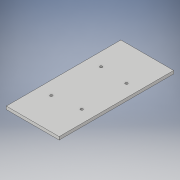
# Autodesk Inventor part: realsenses_plate
Saved by Autodesk Inventor 2019 (Build 230136000, 136)
## iProperties
Created: 2021-06-11
Part Number: realsenses_plate
Material: Типовые
Document SubType Name: Modeling
Designer: Петров Иван
Density: 1 g/cm^3
Appearance: По умолчанию
Author: Петров Иван
Autodesk Inventor part; units mm, degrees
ref_plane "YZ Plane" through (0, 0, 0) normal (1, 0, 0) x (0, 1, 0)
ref_plane "XZ Plane" through (0, 0, 0) normal (0, 1, 0) x (-1, 0, 0)
ref_plane "XY Plane" through (0, 0, 0) normal (0, 0, 1) x (1, 0, 0)
sketch "Sketch1" plane through (0, 0, 0) normal (0, 1, 0) x (-1, 0, 0)
  spline S0 degree 3 poles (-32.404854, -32.853236) (-32.408213, -32.73595) (-32.409911, -32.618547) (-32.409934, -32.501343) (-32.409955, -32.397684) (-32.409974, -32.293904) (-32.409993, -32.190169) (-32.410033, -31.969146) (-32.41007, -31.748122) (-32.410103, -31.527098) (-32.41017, -31.085051) (-32.410223, -30.643004) (-32.410266, -30.200957) (-32.410352, -29.316862) (-32.410395, -28.432768) (-32.410416, -27.548673) (-32.410444, -26.388246) (-32.410435, -25.228046) (-32.410446, -24.067555) (-32.410451, -23.45976) (-32.410462, -22.851867) (-32.410477, -22.244105) (-32.410527, -20.157589) (-32.410619, -18.070753) (-32.410664, -15.984323) (-32.410696, -14.53452) (-32.410704, -13.084832) (-32.410706, -11.63497) (-32.410708, -10.42824) (-32.410705, -9.226696) (-32.410708, -8.025862) (-32.410715, -5.363664) (-32.410749, -2.704993) (-32.410749, 0) (-32.410749, 2.70077) (-32.410715, 5.359553) (-32.410708, 8.025862) (-32.410707, 8.544603) (-32.410707, 9.06363) (-32.410707, 9.583301) (-32.410707, 11.716216) (-32.41071, 13.850051) (-32.410664, 15.984323) (-32.410606, 18.679415) (-32.41047, 21.375766) (-32.410446, 24.067555) (-32.410425, 26.312694) (-32.410471, 28.55511) (-32.410201, 30.801569) (-32.410148, 31.243615) (-32.410083, 31.685661) (-32.410004, 32.127707) (-32.409982, 32.252247) (-32.409959, 32.376902) (-32.409934, 32.501343) (-32.409915, 32.59775) (-32.408764, 32.694267) (-32.406487, 32.790697) (-32.401273, 33.0116) (-32.390165, 33.232367) (-32.373199, 33.452997) (-32.339266, 33.894259) (-32.28153, 34.337158) (-32.200857, 34.773898) (-32.120183, 35.210638) (-32.017096, 35.639812) (-31.892023, 36.061563) (-31.803491, 36.360098) (-31.703903, 36.654969) (-31.593121, 36.94617) (-31.39089, 37.477752) (-31.151562, 37.997105) (-30.875182, 38.502046) (-30.760914, 38.710811) (-30.641216, 38.915391) (-30.516203, 39.115805) (-30.173207, 39.665673) (-29.790661, 40.184302) (-29.36895, 40.672553) (-29.245622, 40.81534) (-29.118935, 40.95548) (-28.988811, 41.092954) (-28.815373, 41.276189) (-28.635833, 41.454691) (-28.450153, 41.628366) (-28.125165, 41.932343) (-27.784487, 42.218481) (-27.432415, 42.483881) (-27.308772, 42.577086) (-27.18357, 42.667861) (-27.056809, 42.756201) (-26.46167, 43.170951) (-25.83254, 43.532746) (-25.16884, 43.840615) (-25.051477, 43.895056) (-24.933051, 43.94777) (-24.813786, 43.998631) (-24.523994, 44.122212) (-24.22923, 44.2348) (-23.933007, 44.33546) (-23.514871, 44.477546) (-23.091358, 44.596955) (-22.662502, 44.693838) (-22.570374, 44.714651) (-22.477996, 44.734419) (-22.38537, 44.753136) (-22.046825, 44.821544) (-21.70496, 44.875937) (-21.359741, 44.916201) (-20.920071, 44.967482) (-20.473811, 44.995783) (-20.027865, 45) knots 0 0 0 0 0.00414579 0.00414579 0.00414579 0.0078125 0.0078125 0.0078125 0.015625 0.015625 0.015625 0.03125 0.03125 0.03125 0.0625 0.0625 0.0625 0.1035175 0.1035175 0.1035175 0.125 0.125 0.125 0.19875187 0.19875187 0.19875187 0.25 0.25 0.25 0.29265414 0.29265414 0.29265414 0.38721651 0.38721651 0.38721651 0.48163124 0.48163124 0.48163124 0.5 0.5 0.5 0.57539191 0.57539191 0.57539191 0.67059447 0.67059447 0.67059447 0.75 0.75 0.75 0.765625 0.765625 0.765625 0.77002712 0.77002712 0.77002712 0.7734375 0.7734375 0.7734375 0.78125 0.78125 0.78125 0.796875 0.796875 0.796875 0.8125 0.8125 0.8125 0.82356007 0.82356007 0.82356007 0.84375 0.84375 0.84375 0.85209742 0.85209742 0.85209742 0.875 0.875 0.875 0.88169776 0.88169776 0.88169776 0.890625 0.890625 0.890625 0.90625 0.90625 0.90625 0.91173731 0.91173731 0.91173731 0.9375 0.9375 0.9375 0.94205566 0.94205566 0.94205566 0.953125 0.953125 0.953125 0.96875 0.96875 0.96875 0.97210662 0.97210662 0.97210662 0.984375 0.984375 0.984375 1 1 1 1
  spline S1 degree 3 poles (-28.410193, 32.5) (-28.410193, 33.765572) (-28.133676, 34.931308) (-27.671254, 35.965522) (-27.208832, 36.999736) (-26.560504, 37.902428) (-25.780808, 38.647111) (-25.001113, 39.391795) (-24.090049, 39.97847) (-23.095481, 40.380521) (-22.100912, 40.782573) (-21.02284, 41) (-19.910193, 41) (-18.797545, 41) (-17.719473, 40.782573) (-16.724904, 40.380521) (-15.730336, 39.97847) (-14.819272, 39.391795) (-14.039577, 38.647111) (-13.259881, 37.902428) (-12.611553, 36.999736) (-12.149131, 35.965522) (-11.686709, 34.931308) (-11.410193, 33.765572) (-11.410193, 32.5) knots 0 0 0 0 0.125 0.125 0.125 0.25 0.25 0.25 0.375 0.375 0.375 0.5 0.5 0.5 0.625 0.625 0.625 0.75 0.75 0.75 0.875 0.875 0.875 1 1 1 1
  line L0 (-28.410193, -32.5) -> (-28.410193, 32.5)
  line L1 (-11.410193, 32.5) -> (-11.410193, -9.130692)
  line L2 (-11.410193, -9.130692) -> (-11.410193, -32.5)
  spline S2 degree 3 poles (-11.92122, -35.403236) (-11.99101, -35.594681) (-12.067149, -35.782168) (-12.149131, -35.965522) (-12.611553, -36.999736) (-13.259881, -37.902428) (-14.039577, -38.647111) (-14.819272, -39.391795) (-15.730336, -39.97847) (-16.724904, -40.380521) (-17.719473, -40.782573) (-18.797545, -41) (-19.910193, -41) (-21.02284, -41) (-22.100912, -40.782573) (-23.095481, -40.380521) (-24.090049, -39.97847) (-25.001113, -39.391795) (-25.780808, -38.647111) (-26.560504, -37.902428) (-27.208832, -36.999736) (-27.671254, -35.965522) (-27.753236, -35.782168) (-27.829375, -35.594681) (-27.899165, -35.403236) knots 0.102839 0.102839 0.102839 0.102839 0.125 0.125 0.125 0.25 0.25 0.25 0.375 0.375 0.375 0.5 0.5 0.5 0.625 0.625 0.625 0.75 0.75 0.75 0.875 0.875 0.875 0.897161 0.897161 0.897161 0.897161
  ellipse E0 centre (-27.409985, -30.903735) end of major axis (-43.224744, -27.538991) minor radius 11.659046 (-11.885471, -35.303236) -> (-11.410193, -32.5) ccw
  ellipse E1 centre (-12.410416, -30.903738) end of major axis (-28.225158, -34.268479) minor radius 11.659041 (-28.410193, -32.5) -> (-27.934914, -35.303236) ccw
  spline S3 degree 3 poles (-20.135916, -44.926171) (-20.902232, -44.912188) (-21.656156, -44.828474) (-22.39639, -44.67772) (-22.948546, -44.56527) (-23.493405, -44.415278) (-24.031365, -44.226793) (-24.310103, -44.129132) (-24.58603, -44.021306) (-24.856048, -43.904514) (-24.890974, -43.889408) (-24.925802, -43.874152) (-24.960525, -43.858751) (-25.263696, -43.724284) (-25.560172, -43.578241) (-25.850131, -43.420931) (-26.291576, -43.181437) (-26.717955, -42.915946) (-27.128881, -42.623661) (-27.257781, -42.531977) (-27.385148, -42.437641) (-27.510974, -42.340653) (-27.774451, -42.137563) (-28.031837, -41.922148) (-28.278086, -41.698847) (-28.524335, -41.475546) (-28.760531, -41.243618) (-28.986777, -41.003148) (-29.015281, -40.972852) (-29.043627, -40.942419) (-29.071813, -40.911851) (-29.491074, -40.457166) (-29.875526, -39.972573) (-30.22442, -39.457475) (-30.348377, -39.274468) (-30.468123, -39.087073) (-30.582688, -38.896485) (-30.640191, -38.800823) (-30.696393, -38.704359) (-30.751212, -38.60729) (-30.915247, -38.316831) (-31.066945, -38.021018) (-31.206902, -37.720112) (-31.358831, -37.393466) (-31.497133, -37.060343) (-31.621381, -36.721723) (-31.726048, -36.436468) (-31.82072, -36.147348) (-31.905041, -35.853236) knots 0 0 0 0 0.14319106 0.14319106 0.14319106 0.25 0.25 0.25 0.30534172 0.30534172 0.30534172 0.3125 0.3125 0.3125 0.375 0.375 0.375 0.47015259 0.47015259 0.47015259 0.5 0.5 0.5 0.5625 0.5625 0.5625 0.625 0.625 0.625 0.63287425 0.63287425 0.63287425 0.75 0.75 0.75 0.7916132 0.7916132 0.7916132 0.8125 0.8125 0.8125 0.875 0.875 0.875 0.94284614 0.94284614 0.94284614 1 1 1 1
  ellipse E2 centre (-27.409985, -30.903735) end of major axis (-43.224744, -27.538991) minor radius 11.659046 (-11.885471, -35.303236) -> (-11.410193, -32.5) ccw
  line L3 (-11.410193, -9.130692) -> (-11.410193, -32.5)
  line L4 (-11.410193, 32.5) -> (-11.410193, -9.130692)
  spline S4 degree 3 poles (-28.410193, 32.5) (-28.410193, 33.765572) (-28.133677, 34.931308) (-27.671254, 35.965522) (-27.208832, 36.999736) (-26.560504, 37.902428) (-25.780809, 38.647111) (-25.001113, 39.391795) (-24.090049, 39.97847) (-23.095481, 40.380521) (-22.100913, 40.782573) (-21.02284, 41) (-19.910193, 41) (-18.797545, 41) (-17.719473, 40.782573) (-16.724904, 40.380521) (-15.730336, 39.97847) (-14.819273, 39.391795) (-14.039577, 38.647111) (-13.259881, 37.902428) (-12.611553, 36.999736) (-12.149131, 35.965522) (-11.686709, 34.931308) (-11.410193, 33.765572) (-11.410193, 32.5) knots 0 0 0 0 0.125 0.125 0.125 0.25 0.25 0.25 0.375 0.375 0.375 0.5 0.5 0.5 0.625 0.625 0.625 0.75 0.75 0.75 0.875 0.875 0.875 1 1 1 1
  line L5 (-28.410193, -32.5) -> (-28.410193, 32.5)
  ellipse E3 centre (-12.410416, -30.903738) end of major axis (-28.225158, -34.268479) minor radius 11.659041 (-28.410193, -32.5) -> (-27.934914, -35.303236) ccw
  circle A0 centre (-19.910193, 22.5) radius 1.25
  circle A1 centre (-19.910193, -22.5) radius 1.25
  spline S5 degree 3 poles (-7.409638, -8.902626) (-7.409642, -11.263271) (-7.409635, -13.623588) (-7.409688, -15.984285) (-7.409726, -17.615445) (-7.409792, -19.246809) (-7.409843, -20.877933) (-7.409877, -21.941017) (-7.409905, -23.004462) (-7.409916, -24.06752) (-7.409926, -25.000298) (-7.409923, -25.932787) (-7.409937, -26.865587) (-7.409952, -27.863529) (-7.409987, -28.861472) (-7.410072, -29.859414) (-7.410115, -30.358385) (-7.410171, -30.857356) (-7.410243, -31.356327) (-7.410279, -31.605813) (-7.410319, -31.855298) (-7.410363, -32.104784) (-7.410387, -32.236971) (-7.410411, -32.369257) (-7.410437, -32.501339) (-7.410461, -32.618544) (-7.412158, -32.735941) (-7.415518, -32.853236) knots 0 0 0 0 0.29568906 0.29568906 0.29568906 0.5 0.5 0.5 0.6331595 0.6331595 0.6331595 0.75 0.75 0.75 0.875 0.875 0.875 0.9375 0.9375 0.9375 0.96875 0.96875 0.96875 0.98530746 0.98530746 0.98530746 1 1 1 1
  spline S6 degree 3 poles (-7.409638, -8.902626) (-7.398668, -9.006825) (-9.14047, -8.698904) (-11.410193, -9.130692) knots 0 0 0 0 1 1 1 1
  line L6 (-11.410193, -9.130692) -> (-11.410193, -32.5)
  ellipse E4 centre (-27.409985, -30.903735) end of major axis (-43.224744, -27.538991) minor radius 11.659046 (-11.885471, -35.303236) -> (-11.410193, -32.5) ccw
  line L7 (-11.885471, -35.303236) -> (-7.757702, -35.303236)
  spline S7 degree 3 poles (-7.757702, -35.303236) (-7.758844, -35.303236) (-7.761073, -35.30773) (-7.767821, -35.325968) (-7.772438, -35.340145) (-7.78659, -35.386369) (-7.797308, -35.423345) (-7.823066, -35.51376) (-7.838041, -35.566981) (-7.866767, -35.668696) (-7.879817, -35.714794) (-7.897842, -35.778081) (-7.902464, -35.794277) (-7.90927, -35.818079) (-7.911434, -35.825641) (-7.915514, -35.839882) (-7.917428, -35.846559) (-7.919345, -35.853236) knots 0 0 0 0 0.13804482 0.13804482 0.28388387 0.28388387 0.50004609 0.50004609 0.72328448 0.72328448 0.89210226 0.89210226 0.94966157 0.94966157 0.97641027 0.97641027 1 1 1 1
  spline S8 degree 3 poles (-7.919345, -35.853236) (-8.003152, -36.145286) (-8.097043, -36.431979) (-8.200582, -36.714498) (-8.328208, -37.062745) (-8.47045, -37.404583) (-8.626747, -37.739075) (-8.810346, -38.131998) (-9.013716, -38.515699) (-9.237855, -38.889015) (-9.35932, -39.09132) (-9.486915, -39.290583) (-9.620818, -39.486955) (-9.811316, -39.766324) (-10.014117, -40.038912) (-10.225707, -40.300477) (-10.393712, -40.508163) (-10.567792, -40.709695) (-10.747887, -40.905165) (-10.794607, -40.955875) (-10.841734, -41.006176) (-10.889261, -41.056069) (-11.350717, -41.540498) (-11.849576, -41.987112) (-12.386918, -42.394816) (-12.486805, -42.470605) (-12.588167, -42.545124) (-12.690734, -42.618124) (-12.864047, -42.741476) (-13.040808, -42.860477) (-13.219487, -42.974259) (-13.503909, -43.155378) (-13.7942, -43.324035) (-14.090213, -43.480544) (-14.376118, -43.631709) (-14.667362, -43.771537) (-14.964004, -43.8999) (-15.281618, -44.037338) (-15.605429, -44.161639) (-15.935451, -44.272737) (-16.254577, -44.380167) (-16.581053, -44.475594) (-16.9089, -44.557066) (-17.080253, -44.599649) (-17.251997, -44.638463) (-17.424125, -44.673526) (-17.581326, -44.705549) (-17.738847, -44.734442) (-17.896686, -44.760264) (-18.558021, -44.868455) (-19.224843, -44.923373) (-19.897251, -44.924079) (-19.901566, -44.924083) (-19.90588, -44.924086) (-19.910193, -44.924086) (-20.241963, -44.924086) (-20.576611, -44.910627) (-20.909693, -44.883796) (-21.247106, -44.856615) (-21.5813, -44.815961) (-21.912343, -44.762119) (-22.074408, -44.73576) (-22.235717, -44.706233) (-22.39627, -44.673528) (-22.891627, -44.572622) (-23.379775, -44.441685) (-23.860799, -44.280846) (-24.196316, -44.16866) (-24.529506, -44.041364) (-24.856421, -43.899904) (-25.150109, -43.772821) (-25.438729, -43.634322) (-25.719775, -43.486069) (-26.209658, -43.227655) (-26.679695, -42.938431) (-27.129738, -42.618131) (-27.225287, -42.550128) (-27.319927, -42.480713) (-27.41366, -42.409893) (-27.948886, -42.0055) (-28.458682, -41.551215) (-28.922894, -41.064862) (-28.973321, -41.01203) (-29.02324, -40.9588) (-29.072649, -40.905176) (-29.478082, -40.465148) (-29.849491, -39.998649) (-30.186959, -39.505722) (-30.324635, -39.304624) (-30.456615, -39.099116) (-30.58276, -38.889029) (-30.630057, -38.810259) (-30.676532, -38.730845) (-30.722184, -38.6508) (-30.889595, -38.357265) (-31.045877, -38.05518) (-31.189193, -37.749189) (-31.347794, -37.410564) (-31.491558, -37.065293) (-31.620128, -36.714515) (-31.723916, -36.431349) (-31.817776, -36.144633) (-31.901409, -35.853236) knots 0 0 0 0 0.02799367 0.02799367 0.02799367 0.0625 0.0625 0.0625 0.10303401 0.10303401 0.10303401 0.125 0.125 0.125 0.15625 0.15625 0.15625 0.18106293 0.18106293 0.18106293 0.1875 0.1875 0.1875 0.25 0.25 0.25 0.26161819 0.26161819 0.26161819 0.28125 0.28125 0.28125 0.3125 0.3125 0.3125 0.34268303 0.34268303 0.34268303 0.375 0.375 0.375 0.40625 0.40625 0.40625 0.42258324 0.42258324 0.42258324 0.4375 0.4375 0.4375 0.5 0.5 0.5 0.50040103 0.50040103 0.50040103 0.53125 0.53125 0.53125 0.5625 0.5625 0.5625 0.57779868 0.57779868 0.57779868 0.625 0.625 0.625 0.65792316 0.65792316 0.65792316 0.6875 0.6875 0.6875 0.7390545 0.7390545 0.7390545 0.75 0.75 0.75 0.8125 0.8125 0.8125 0.81928929 0.81928929 0.81928929 0.875 0.875 0.875 0.89772826 0.89772826 0.89772826 0.90625 0.90625 0.90625 0.9375 0.9375 0.9375 0.97208291 0.97208291 0.97208291 1 1 1 1
  spline S9 degree 3 poles (-31.901409, -35.853236) (-31.903324, -35.846565) (-31.905236, -35.839895) (-31.909312, -35.82567) (-31.911474, -35.818117) (-31.918271, -35.79435) (-31.922886, -35.778181) (-31.940872, -35.715036) (-31.953892, -35.669047) (-31.982604, -35.567376) (-31.997591, -35.514102) (-32.023361, -35.423609) (-32.034081, -35.386601) (-32.048248, -35.340272) (-32.052873, -35.326045) (-32.05963, -35.307745) (-32.061857, -35.303236) (-32.062995, -35.303236) knots 0 0 0 0 0.02356692 0.02356692 0.05028405 0.05028405 0.10774901 0.10774901 0.27614786 0.27614786 0.49948807 0.49948807 0.71561552 0.71561552 0.86172473 0.86172473 1 1 1 1
  line L8 (-32.062995, -35.303236) -> (-27.934914, -35.303236)
  ellipse E5 centre (-12.410416, -30.903738) end of major axis (-28.225158, -34.268479) minor radius 11.659041 (-28.410193, -32.5) -> (-27.934914, -35.303236) ccw
  line L9 (-28.410193, -32.5) -> (-28.410193, 32.5)
  spline S10 degree 3 poles (-28.410193, 32.5) (-28.410193, 33.765572) (-28.133676, 34.931308) (-27.671254, 35.965522) (-27.208832, 36.999736) (-26.560504, 37.902428) (-25.780808, 38.647111) (-25.001113, 39.391795) (-24.090049, 39.97847) (-23.095481, 40.380521) (-22.100912, 40.782573) (-21.02284, 41) (-19.910193, 41) (-18.797545, 41) (-17.719473, 40.782573) (-16.724904, 40.380521) (-15.730336, 39.97847) (-14.819272, 39.391795) (-14.039577, 38.647111) (-13.259881, 37.902428) (-12.611553, 36.999736) (-12.149131, 35.965522) (-11.686709, 34.931308) (-11.410193, 33.765572) (-11.410193, 32.5) knots 0 0 0 0 0.125 0.125 0.125 0.25 0.25 0.25 0.375 0.375 0.375 0.5 0.5 0.5 0.625 0.625 0.625 0.75 0.75 0.75 0.875 0.875 0.875 1 1 1 1
  line L10 (-11.410193, 32.5) -> (-11.410193, -9.130692)
  spline S11 degree 3 poles (-7.409638, -8.902626) (-7.408932, -8.899194) (-7.41554, -8.881327) (-7.442844, -8.816766) (-7.463738, -8.769717) (-7.536437, -8.603714) (-7.599257, -8.458754) (-7.724577, -8.122213) (-7.786434, -7.935427) (-7.879306, -7.556662) (-7.913159, -7.371174) (-7.937278, -7.119769) (-7.941464, -7.06115) (-7.945382, -6.9757) (-7.946297, -6.949166) (-7.947438, -6.899489) (-7.947739, -6.876366) (-7.947807, -6.853236) knots 0 0 0 0 0.13056971 0.13056971 0.2645065 0.2645065 0.49982844 0.49982844 0.71627112 0.71627112 0.89885892 0.89885892 0.95382194 0.95382194 0.9785172 0.9785172 1 1 1 1
  spline S12 degree 3 poles (-7.947807, -6.853236) (-7.954633, -4.568884) (-7.957468, -2.286953) (-7.957468, 0) (-7.957468, 2.385018) (-7.954386, 4.76446) (-7.946908, 7.146764) knots 0 0 0 0 0.48950496 0.48950496 0.48950496 1 1 1 1
  spline S13 degree 3 poles (-7.946908, 7.146764) (-7.946835, 7.169899) (-7.946531, 7.193028) (-7.945383, 7.242716) (-7.944465, 7.269255) (-7.940538, 7.354723) (-7.936347, 7.413355) (-7.912212, 7.66482) (-7.878365, 7.850357) (-7.785562, 8.229172) (-7.723783, 8.415967) (-7.598689, 8.752471) (-7.536024, 8.897388) (-7.46354, 9.063319) (-7.442718, 9.110341) (-7.415511, 9.174866) (-7.408931, 9.192724) (-7.409638, 9.196154) knots 0 0 0 0 0.02148885 0.02148885 0.04619107 0.04619107 0.10116958 0.10116958 0.28381522 0.28381522 0.50028176 0.50028176 0.73556793 0.73556793 0.86946283 0.86946283 1 1 1 1
  ellipse E6 centre (-19.910191, 45) end of major axis (-20.032475, 45) minor radius 0 (-20.027865, 45) -> (-19.792521, 45) ccw
  spline S14 degree 3 poles (-32.404854, -32.853236) (-32.408213, -32.73595) (-32.409911, -32.618547) (-32.409934, -32.501343) (-32.409955, -32.397684) (-32.409974, -32.293904) (-32.409993, -32.190169) (-32.410033, -31.969146) (-32.41007, -31.748122) (-32.410103, -31.527098) (-32.41017, -31.085051) (-32.410223, -30.643004) (-32.410266, -30.200957) (-32.410352, -29.316862) (-32.410395, -28.432768) (-32.410416, -27.548673) (-32.410444, -26.388246) (-32.410435, -25.228046) (-32.410446, -24.067555) (-32.410451, -23.45976) (-32.410462, -22.851867) (-32.410477, -22.244105) (-32.410527, -20.157589) (-32.410619, -18.070753) (-32.410664, -15.984323) (-32.410696, -14.53452) (-32.410704, -13.084832) (-32.410706, -11.63497) (-32.410708, -10.42824) (-32.410705, -9.226696) (-32.410708, -8.025862) (-32.410715, -5.363664) (-32.410749, -2.704993) (-32.410749, 0) (-32.410749, 2.70077) (-32.410715, 5.359553) (-32.410708, 8.025862) (-32.410707, 8.544603) (-32.410707, 9.06363) (-32.410707, 9.583301) (-32.410707, 11.716216) (-32.41071, 13.850051) (-32.410664, 15.984323) (-32.410606, 18.679415) (-32.41047, 21.375766) (-32.410446, 24.067555) (-32.410425, 26.312694) (-32.410471, 28.55511) (-32.410201, 30.801569) (-32.410148, 31.243615) (-32.410083, 31.685661) (-32.410004, 32.127707) (-32.409982, 32.252247) (-32.409959, 32.376902) (-32.409934, 32.501343) (-32.409915, 32.59775) (-32.408764, 32.694267) (-32.406487, 32.790697) (-32.401273, 33.0116) (-32.390165, 33.232367) (-32.373199, 33.452997) (-32.339266, 33.894259) (-32.28153, 34.337158) (-32.200857, 34.773898) (-32.120183, 35.210638) (-32.017096, 35.639812) (-31.892023, 36.061563) (-31.803491, 36.360098) (-31.703903, 36.654969) (-31.593121, 36.94617) (-31.39089, 37.477752) (-31.151562, 37.997105) (-30.875182, 38.502046) (-30.760914, 38.710811) (-30.641216, 38.915391) (-30.516203, 39.115805) (-30.173207, 39.665673) (-29.790661, 40.184302) (-29.36895, 40.672553) (-29.245622, 40.81534) (-29.118935, 40.95548) (-28.988811, 41.092954) (-28.815373, 41.276189) (-28.635833, 41.454691) (-28.450153, 41.628366) (-28.125165, 41.932343) (-27.784487, 42.218481) (-27.432415, 42.483881) (-27.308772, 42.577086) (-27.18357, 42.667861) (-27.056809, 42.756201) (-26.46167, 43.170951) (-25.83254, 43.532746) (-25.16884, 43.840615) (-25.051477, 43.895056) (-24.933051, 43.94777) (-24.813786, 43.998631) (-24.523994, 44.122212) (-24.22923, 44.2348) (-23.933007, 44.33546) (-23.514871, 44.477546) (-23.091358, 44.596955) (-22.662502, 44.693838) (-22.570374, 44.714651) (-22.477996, 44.734419) (-22.38537, 44.753136) (-22.046825, 44.821544) (-21.70496, 44.875937) (-21.359741, 44.916201) (-20.920071, 44.967482) (-20.473811, 44.995783) (-20.027865, 45) knots 0 0 0 0 0.00414579 0.00414579 0.00414579 0.0078125 0.0078125 0.0078125 0.015625 0.015625 0.015625 0.03125 0.03125 0.03125 0.0625 0.0625 0.0625 0.1035175 0.1035175 0.1035175 0.125 0.125 0.125 0.19875187 0.19875187 0.19875187 0.25 0.25 0.25 0.29265414 0.29265414 0.29265414 0.38721651 0.38721651 0.38721651 0.48163124 0.48163124 0.48163124 0.5 0.5 0.5 0.57539191 0.57539191 0.57539191 0.67059447 0.67059447 0.67059447 0.75 0.75 0.75 0.765625 0.765625 0.765625 0.77002712 0.77002712 0.77002712 0.7734375 0.7734375 0.7734375 0.78125 0.78125 0.78125 0.796875 0.796875 0.796875 0.8125 0.8125 0.8125 0.82356007 0.82356007 0.82356007 0.84375 0.84375 0.84375 0.85209742 0.85209742 0.85209742 0.875 0.875 0.875 0.88169776 0.88169776 0.88169776 0.890625 0.890625 0.890625 0.90625 0.90625 0.90625 0.91173731 0.91173731 0.91173731 0.9375 0.9375 0.9375 0.94205566 0.94205566 0.94205566 0.953125 0.953125 0.953125 0.96875 0.96875 0.96875 0.97210662 0.97210662 0.97210662 0.984375 0.984375 0.984375 1 1 1 1
  spline S15 degree 3 poles (-32.326118, -33.903236) (-32.327007, -33.903236) (-32.328715, -33.895) (-32.333743, -33.861541) (-32.337123, -33.835589) (-32.347083, -33.749915) (-32.354346, -33.680402) (-32.369383, -33.51231) (-32.377025, -33.415241) (-32.389523, -33.2211) (-32.394565, -33.12798) (-32.399896, -33.000336) (-32.401115, -32.968405) (-32.402735, -32.921618) (-32.403222, -32.906877) (-32.404093, -32.879166) (-32.404483, -32.866202) (-32.404854, -32.853236) knots 0 0 0 0 0.13773636 0.13773636 0.28245528 0.28245528 0.4998262 0.4998262 0.71460149 0.71460149 0.89132086 0.89132086 0.94969153 0.94969153 0.97647884 0.97647884 1 1 1 1
  line L11 (-32.275001, -33.903236) -> (-32.326118, -33.903236)
  spline S16 degree 3 poles (-32.082303, -34.853236) (-32.084676, -34.841371) (-32.087042, -34.829506) (-32.09207, -34.804213) (-32.094728, -34.790789) (-32.103063, -34.748561) (-32.108688, -34.719844) (-32.130326, -34.608554) (-32.145652, -34.527896) (-32.178504, -34.352726) (-32.195119, -34.262366) (-32.224113, -34.107828) (-32.236352, -34.04447) (-32.25334, -33.965771) (-32.25917, -33.941768) (-32.268606, -33.91085) (-32.272281, -33.903236) (-32.275001, -33.903236) knots 0 0 0 0 0.02405151 0.02405151 0.0512956 0.0512956 0.10987642 0.10987642 0.27988487 0.27988487 0.49965886 0.49965886 0.71628377 0.71628377 0.86179308 0.86179308 1 1 1 1
  spline S17 degree 3 poles (-20.17139, -44.853236) (-20.878029, -44.838222) (-21.573226, -44.763643) (-22.257416, -44.631762) (-22.301762, -44.623215) (-22.346062, -44.614422) (-22.390317, -44.605384) (-23.028853, -44.474979) (-23.65793, -44.294096) (-24.276424, -44.061427) (-24.47081, -43.988301) (-24.66254, -43.910608) (-24.851638, -43.828396) (-25.305911, -43.630899) (-25.745054, -43.407502) (-26.16963, -43.159057) (-26.497285, -42.967327) (-26.816345, -42.760565) (-27.126353, -42.538413) (-27.385274, -42.35287) (-27.637877, -42.156573) (-27.883918, -41.949598) (-28.305343, -41.595087) (-28.698989, -41.216742) (-29.065485, -40.815445) (-29.16915, -40.701936) (-29.270623, -40.586577) (-29.369939, -40.469336) (-29.811526, -39.948054) (-30.211115, -39.389501) (-30.564084, -38.794047) (-30.571157, -38.782114) (-30.578212, -38.770167) (-30.585247, -38.758206) (-30.943356, -38.149318) (-31.244219, -37.518322) (-31.494339, -36.86773) (-31.525136, -36.787624) (-31.555162, -36.707173) (-31.584396, -36.626428) (-31.792589, -36.051387) (-31.960654, -35.461445) (-32.082303, -34.853236) knots 0 0 0 0 0.125 0.125 0.125 0.13310181 0.13310181 0.13310181 0.25 0.25 0.25 0.28673977 0.28673977 0.28673977 0.375 0.375 0.375 0.44311226 0.44311226 0.44311226 0.5 0.5 0.5 0.5974389 0.5974389 0.5974389 0.625 0.625 0.625 0.74754435 0.74754435 0.74754435 0.75 0.75 0.75 0.875 0.875 0.875 0.89039091 0.89039091 0.89039091 1 1 1 1
  line L12 (-20.17139, -44.853236) -> (-19.649008, -44.853236)
  spline S18 degree 3 poles (-7.738713, -34.853236) (-7.860311, -35.461404) (-8.028327, -36.051343) (-8.236488, -36.626409) (-8.265735, -36.707207) (-8.295776, -36.787711) (-8.326589, -36.867869) (-8.576705, -37.518543) (-8.877592, -38.149652) (-9.235782, -38.758677) (-9.242721, -38.770476) (-9.249678, -38.78226) (-9.256654, -38.79403) (-9.609761, -39.389781) (-10.009148, -39.948038) (-10.450617, -40.469231) (-10.549953, -40.586506) (-10.651446, -40.701897) (-10.755129, -40.815433) (-11.121335, -41.21644) (-11.514619, -41.594489) (-11.935591, -41.948716) (-12.181737, -42.155836) (-12.434737, -42.352496) (-12.69416, -42.538407) (-13.004032, -42.760472) (-13.323062, -42.967221) (-13.650378, -43.158779) (-14.075179, -43.40739) (-14.514473, -43.63087) (-14.9688, -43.828397) (-15.15761, -43.910486) (-15.349026, -43.988062) (-15.543071, -44.06108) (-16.161281, -44.293705) (-16.791217, -44.474918) (-17.430074, -44.605391) (-17.47426, -44.614415) (-17.518489, -44.623194) (-17.562759, -44.631729) (-18.247107, -44.763656) (-18.942379, -44.838234) (-19.649008, -44.853236) knots 0 0 0 0 0.10960083 0.10960083 0.10960083 0.125 0.125 0.125 0.25 0.25 0.25 0.25242164 0.25242164 0.25242164 0.375 0.375 0.375 0.4025818 0.4025818 0.4025818 0.5 0.5 0.5 0.55696145 0.55696145 0.55696145 0.625 0.625 0.625 0.71330281 0.71330281 0.71330281 0.75 0.75 0.75 0.86691377 0.86691377 0.86691377 0.875 0.875 0.875 1 1 1 1
  spline S19 degree 3 poles (-7.545928, -33.903236) (-7.548655, -33.903236) (-7.552333, -33.910824) (-7.561767, -33.941634) (-7.567592, -33.965551) (-7.584574, -34.044068) (-7.596815, -34.10737) (-7.625801, -34.261778) (-7.642403, -34.352049) (-7.675265, -34.527294) (-7.690621, -34.608135) (-7.712301, -34.719667) (-7.717932, -34.748431) (-7.726277, -34.790723) (-7.728938, -34.804162) (-7.733969, -34.829483) (-7.736337, -34.84136) (-7.738713, -34.853236) knots 0 0 0 0 0.13797105 0.13797105 0.28320611 0.28320611 0.49987241 0.49987241 0.71955484 0.71955484 0.88997298 0.88997298 0.94864929 0.94864929 0.97592532 0.97592532 1 1 1 1
  line L13 (-7.494451, -33.903236) -> (-7.545928, -33.903236)
  spline S20 degree 3 poles (-7.415518, -32.853236) (-7.415889, -32.866192) (-7.416279, -32.879146) (-7.417149, -32.906834) (-7.417636, -32.921561) (-7.419255, -32.968293) (-7.420473, -33.000185) (-7.425797, -33.127573) (-7.43083, -33.220493) (-7.443328, -33.414553) (-7.450985, -33.51171) (-7.466057, -33.679936) (-7.47334, -33.749507) (-7.483349, -33.835367) (-7.486752, -33.861406) (-7.491821, -33.894974) (-7.493547, -33.903236) (-7.494451, -33.903236) knots 0 0 0 0 0.02350348 0.02350348 0.05026558 0.05026558 0.10856122 0.10856122 0.28487722 0.28487722 0.49973499 0.49973499 0.71707093 0.71707093 0.86204486 0.86204486 1 1 1 1
  circle A2 centre (7.26, 25.808503) radius 1.2645
  circle A3 centre (7.26, -24.191497) radius 1.2645
  line L14 (14.52, 49.818503) -> (14.52, -48.201497)
  line L15 (14.52, -48.201497) -> (0, -48.201497)
  line L16 (0, -48.201497) -> (0, 49.818503)
  line L17 (0, 49.818503) -> (14.52, 49.818503)
  arc A4 (0.01, 54.808503) -> (-4.99, 49.808503) centre (0.01, 49.808503) ccw
  arc A5 (0.01, 54.808503) -> (-4.99, 49.808503) centre (0.01, 49.808503) ccw
  line L18 (-4.99, 49.808503) -> (-4.99, -48.191497)
  arc A6 (-4.99, -48.191497) -> (0.01, -53.191497) centre (0.01, -48.191497) ccw
  line L19 (0.01, -53.191497) -> (14.51, -53.191497)
  arc A7 (14.51, -53.191497) -> (19.51, -48.191497) centre (14.51, -48.191497) ccw
  line L20 (19.51, -48.191497) -> (19.51, 49.808503)
  arc A8 (19.51, 49.808503) -> (14.51, 54.808503) centre (14.51, 49.808503) ccw
  line L21 (14.51, 54.808503) -> (0.01, 54.808503)
  line L22 (0, 54.308503) -> (14.52, 54.308503)
  arc A9 (19.01, 49.818503) -> (14.52, 54.308503) centre (14.52, 49.818503) ccw
  line L23 (19.01, 49.818503) -> (19.01, -48.201497)
  arc A10 (14.52, -52.691497) -> (19.01, -48.201497) centre (14.52, -48.201497) ccw
  line L24 (14.52, -52.691497) -> (0, -52.691497)
  arc A11 (-4.49, -48.201497) -> (0, -52.691497) centre (0, -48.201497) ccw
  line L25 (-4.49, -48.201497) -> (-4.49, 49.818503)
  arc A12 (0, 54.308503) -> (-4.49, 49.818503) centre (0, 49.818503) ccw
  line L26 (-32.359548, 57.565226) -> (20.681148, 57.565226)
  line L27 (20.681148, 57.565226) -> (20.681148, -57.434774)
  line L28 (20.681148, -57.434774) -> (-32.359548, -57.434774)
  line L29 (-32.359548, -57.434774) -> (-32.359548, 57.565226)
  point P0 (0, 0)
  point P1 (-19.910193, 0)
  point P2 (6.940853, 0.065226)
  point P3 (2.640452, 0.065226)
  dimension "d1" = 115
  constraints: 60 end point, 18 point on circle, 13 centre point, 2 parallel, 1 horizontal, 1 perpendicular, 72 other
  measures "d1" distance of L26.end L27.end
sketch "Sketch1 outline for Extrusion1" plane through (0, 0, 0) normal (0, 1, 0) x (-1, 0, 0)
  line L0 (-32.359548, 57.565226) -> (20.681148, 57.565226)
  line L1 (-32.359548, -57.434774) -> (-32.359548, 57.565226)
  line L2 (20.681148, 57.565226) -> (20.681148, -57.434774)
  line L3 (20.681148, -57.434774) -> (-32.359548, -57.434774)
  circle A0 centre (-19.910193, -22.5) radius 1.25
  circle A1 centre (7.26, -24.191497) radius 1.2645
  circle A2 centre (-19.910193, 22.5) radius 1.25
  circle A3 centre (7.26, 25.808503) radius 1.2645
extrude "Extrusion1" add sketch "Sketch1 outline for Extrusion1" along normal blind 3
body "Solid1"
